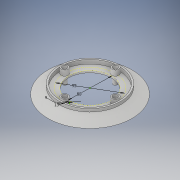
# Autodesk Inventor part: BaseHumedadDireccion
Saved by Autodesk Inventor 2019 (Build 230136000, 136)
## iProperties
Created: 2020-03-30
Part Number: BaseHumedadDireccion
Material: Generic
Document SubType Name: Modeling
Designer: Sergio
Density: 1 g/cm^3
Appearance: Default
Author: Sergio
Autodesk Inventor part; units mm, degrees
ref_plane "YZ Plane" through (0, 0, 0) normal (1, 0, 0) x (0, 1, 0)
ref_plane "XZ Plane" through (0, 0, 0) normal (0, 1, 0) x (-1, 0, 0)
ref_plane "XY Plane" through (0, 0, 0) normal (0, 0, 1) x (1, 0, 0)
sketch "Sketch1" plane through (0, 0, 0) normal (0, 1, 0) x (-1, 0, 0)
  circle A0 centre (0, 0) radius 55
  dimension "d4" = 110
  constraints: 1 centre point
  measures "d4" diameter of A0
sketch "Sketch2" plane through (0, 0, 0) normal (0, 1, 0) x (-1, 0, 0)
  circle A0 centre (0, 0) radius 40 construction
  circle A1 centre (0, 0) radius 47.5 construction
  circle A2 centre (0, 47.5) radius 4.5
  circle A3 centre (0, 47.5) radius 6.5
  dimension "d11" = 95
  dimension "d10" = 80
  dimension "d12" = 9
  dimension "d13" = 13
  constraints: 3 centre point, 3 coincident, 1 vertical alignment, 2 other
  measures "d10" diameter of A0
  measures "d12" diameter of A2
  measures "d13" diameter of A3
extrude "Extrusion1" add sketch "Sketch1" against normal blind 3.5
extrude "Extrusion2" add sketch "Sketch2" along normal blind 10
pattern_circular "Circular Pattern1" count 4 over 360 about axis through (0, -10, 0) along (0, 1, 0) of "Extrusion2"
sketch "Sketch3" plane through (0, -3.5, 0) normal (0, -1, 0) x (1, 0, 0)
  circle A0 centre (0, 0) radius 55
  circle A1 centre (0, 0) radius 55 projected
  circle A2 centre (0, 0) radius 58
  dimension "d21" = 116
  constraints: 2 centre point, 2 coincident, 1 concentric
  measures "d21" diameter of A2
extrude "Extrusion3" add sketch "Sketch3" against normal blind 11
sketch "Sketch4" plane through (0, 0, 0) normal (0, 1, 0) x (1, 0, 0)
  circle A0 centre (0, 0) radius 40
  dimension "d24" = 80
  constraints: 1 centre point, 1 coincident
  measures "d24" diameter of A0
extrude "Extrusion4" cut sketch "Sketch4" against normal blind 30
sketch "Sketch5" plane through (0, 0, 0) normal (0, 0, 1) x (1, 0, 0)
  line L0 (58, -3.5) -> (-58, -3.5) projected
  line L1 (-58, 2) -> (-78.7846, -10)
  line L2 (-76.2846, -10) -> (-58, -3.5)
  line L3 (-58, -3.5) -> (-58, 2)
  line L4 (-105.5118, 0) -> (85.252, 0) projected
  line L5 (-78.7846, -10) -> (-76.2846, -10)
  line L6 (0, -22.2) -> (0, 3.7) projected
  point P0 (0, 0)
  dimension "d29" = 30
  dimension "d30" = 12
  dimension "d32" = 2.5
  dimension "d33" = 5.5
  dimension "d42" = 20.7846
  constraints: 8 end point, 1 horizontal, 1 parallel, 1 perpendicular
  measures "d29" angle of L4 L1
  measures "d30" vertical distance of L1.start L1.end
  measures "d32" distance of L1.end L2.start
  measures "d33" distance of L0.end L1.start
  measures "d42" horizontal distance of L1.start L1.end
revolve "Revolution1" add sketch "Sketch5" angle 360 about axis through (0, -10, 0) along (0, 1, 0) contours L2 L5 L1 L4 L3 | L4 L1 L3
sketch "Sketch6" plane through (0, -3.5, 0) normal (0, -1, 0) x (1, 0, 0)
  circle A0 centre (0, 0) radius 47.5 construction
  circle A1 centre (0, 47.5) radius 6.5 projected
  circle A2 centre (0, 47.5) radius 4
  dimension "d35" = 95
  dimension "d36" = 8
  constraints: 2 centre point, 2 coincident
  measures "d35" diameter of A0
  measures "d36" diameter of A2
extrude "Extrusion5" add sketch "Sketch6" along normal blind 13 contours A2
pattern_circular "Circular Pattern2" count 4 over 360 about axis through (0, 0, 0) along (0, -1, 0) of "Extrusion5"
body "Solid1"
